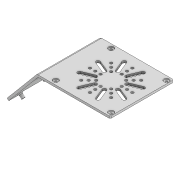
# Autodesk Inventor part: Electronics holder
Saved by Autodesk Inventor 2020 (Build 240168000, 168)
## iProperties
Created: 2021-10-18
Part Number: Electronics holder
Material: Generic
Document SubType Name: Modeling
Designer: ferrerx
Density: 1 g/cm^3
Appearance: Default
Author: ferrerx
Autodesk Inventor part; units mm, degrees
ref_plane "YZ Plane" through (0, 0, 0) normal (1, 0, 0) x (0, 1, 0)
ref_plane "XZ Plane" through (0, 0, 0) normal (0, 1, 0) x (-1, 0, 0)
sketch "Sketch1" plane through (0, 0, 0) normal (0, 1, 0) x (-1, 0, 0)
  line L0 (-52.25, 52.25) -> (52.25, 52.25) construction
  line L1 (52.25, 52.25) -> (52.25, -52.25) construction
  line L2 (52.25, -52.25) -> (-52.25, -52.25) construction
  line L3 (-52.25, -52.25) -> (-52.25, 52.25) construction
  line L4 (-52.25, 52.25) -> (52.25, -52.25) construction
  line L5 (52.25, 52.25) -> (-52.25, -52.25) construction
  line L6 (-80, 60) -> (80, 60)
  line L7 (80, 60) -> (80, -60)
  line L8 (80, -60) -> (-80, -60)
  line L9 (-80, -60) -> (-80, 60)
  line L10 (-80, 60) -> (80, -60) construction
  line L11 (80, 60) -> (-80, -60) construction
  circle A0 centre (52.25, 52.25) radius 2
  circle A1 centre (52.25, -52.25) radius 2
  circle A2 centre (-52.25, -52.25) radius 2
  circle A3 centre (-52.25, 52.25) radius 2
  point P0 (0, 0)
  dimension "d0" = 104.5
  dimension "d1" = 104.5
  dimension "d2" = 160
  dimension "d3" = 120
  dimension "d4" = 4
  dimension "d5" = 4
  dimension "d6" = 4
  dimension "d7" = 4
  constraints: 24 end point, 4 centre point, 4 coincident, 4 midpoint, 4 parallel, 2 horizontal, 2 perpendicular
  measures "d0" distance of L1.end L2.end
  measures "d1" distance of L0.end L1.end
  measures "d2" distance of L7.end L8.end
  measures "d3" distance of L6.end L7.end
  measures "d4" diameter of A0
  measures "d5" diameter of A1
  measures "d6" diameter of A3
  measures "d7" diameter of A2
extrude "Extrusion1" add sketch "Sketch1" along normal blind 4
sketch "Sketch2" plane through (0, 4, 0) normal (0, 1, 0) x (1, 0, 0)
  line L0 (-43.10961, -50) -> (-39.10961, -50)
  line L1 (-39.10961, -50) -> (-39.10961, 50)
  line L2 (-39.10961, 50) -> (-43.10961, 50)
  line L3 (-43.10961, 50) -> (-43.10961, -50)
  line L4 (-43.10961, -50) -> (-39.10961, 50) construction
  line L5 (-39.10961, -50) -> (-43.10961, 50) construction
  line L6 (0, 0) -> (-41.10961, 0) construction
  dimension "d10" = 4
  dimension "d11" = 100
  constraints: 14 end point, 2 horizontal, 2 midpoint, 2 parallel, 1 perpendicular
  measures "d10" distance of L1.end L2.end
  measures "d11" distance of L2.end L0.start
extrude "Extrusion2" [suppressed]
sketch "Sketch3" plane through (0, 4, 0) normal (0, 1, 0) x (1, 0, 0)
  circle A0 centre (0, 0) radius 2.5
  dimension "d14" = 5
  constraints: 1 centre point, 1 coincident
  measures "d14" diameter of A0
extrude "Extrusion3" cut sketch "Sketch3" against normal blind 4
pattern_linear "Rectangular Pattern1" count 5 spacing 10 along (1, 0, 0) of "Extrusion3"
pattern_circular "Circular Pattern1" count 8 over 360 about axis through (0, 4, 0) along (0, -1, 0) of "Extrusion3", "Rectangular Pattern1"
sketch "Sketch4" plane through (0, 4, 0) normal (0, 1, 0) x (1, 0, 0)
  line L0 (0, 0) -> (-19.859021, 47.943918) construction
  circle A0 centre (0, 0) radius 2.5
  line L1 (0, 0) -> (0, 50) construction
  line L2 (-8.905592, 21.5) -> (-17.604076, 42.5) construction
  line L3 (-5.672013, 22.839392) -> (-14.370498, 43.839392)
  line L4 (-20.837655, 41.160608) -> (-12.13917, 20.160608)
  arc A1 (-12.13917, 20.160608) -> (-5.672013, 22.839392) centre (-8.905592, 21.5) ccw
  arc A2 (-14.370498, 43.839392) -> (-20.837655, 41.160608) centre (-17.604076, 42.5) ccw
  point P0 (-13.254834, 32)
  dimension "d23" = 22.5
  dimension "d24" = 32
  dimension "d94" = 7
  constraints: 12 end point, 4 point on circle, 4 tangent, 2 centre point, 2 point on line, 1 midpoint, 1 parallel, 1 vertical
  measures "d23" angle of L0 L1
  measures "d24" vertical distance of L0.start point (-13.255, 32)
  measures "d94" distance between parallel lines of L4 L3
extrude "Extrusion4" cut sketch "Sketch4" against normal blind 4 contours A1 L4 A2 L3
pattern_circular "Circular Pattern2" count 8 over 360 about axis through (0, 4, 0) along (0, -1, 0) of "Extrusion4"
ref_plane "Work Plane1" through (-80, 4, -60) normal (0.7660444, -0.6427876, 0) x (0, 0, 1)
sketch "Sketch5" plane through (-80, 4, -60) normal (0.7660444, -0.6427876, 0) x (0, 0, 1)
  line L0 (1.217722, 0) -> (120, 0)
  line L1 (120, 0) -> (0, 0)
  line L2 (0, 0) -> (0, 90)
  line L3 (0, 90) -> (120, 90)
  line L4 (120, 90) -> (120, 0)
  line L5 (0, -102.846018) -> (0, 0)
  line L6 (0, 0) -> (120, 0)
  point P0 (60, -48.358831)
  point P1 (0, 2.294306)
  dimension "d31" = 90
  constraints: 10 end point, 2 collinear, 2 parallel, 1 horizontal, 1 perpendicular
  measures "d31" distance of L1.end L2.end
extrude "Extrusion5" add sketch "Sketch5" along normal blind 4
sketch "Sketch6" plane through (-80, 4, -60) normal (-0.7660444, 0.6427876, 0) x (0, 0, 1)
  line L0 (0, 0) -> (120, 0) projected
  line L1 (60, 0) -> (60, -90) construction
  line L2 (105, -12.5) -> (15, -12.5) construction
  line L3 (15, -12.5) -> (15, -77.5) construction
  line L4 (15, -77.5) -> (105, -77.5) construction
  line L5 (105, -77.5) -> (105, -12.5) construction
  line L6 (105, -12.5) -> (15, -77.5) construction
  line L7 (15, -12.5) -> (105, -77.5) construction
  circle A0 centre (105, -77.5) radius 1.5
  circle A1 centre (105, -12.5) radius 1.5
  circle A2 centre (15, -12.5) radius 1.5
  circle A3 centre (15, -77.5) radius 1.5
  point P0 (60, 48.358831)
  point P1 (60, -45)
  dimension "d34" = 65
  dimension "d35" = 90
  dimension "d36" = 3
  dimension "d37" = 3
  dimension "d38" = 3
  dimension "d39" = 3
  constraints: 14 end point, 4 centre point, 4 coincident, 4 midpoint, 2 parallel, 1 horizontal, 1 perpendicular, 1 vertical
  measures "d34" distance of L2.end L3.end
  measures "d35" distance of L2.start L2.end
  measures "d36" diameter of A3
  measures "d37" diameter of A2
  measures "d38" diameter of A1
  measures "d39" diameter of A0
extrude "Extrusion6" cut sketch "Sketch6" against normal blind 4
sketch "Sketch7" plane through (-80, 4, -60) normal (-0.7660444, 0.6427876, 0) x (0, 0, 1)
  line L0 (71.5, -36) -> (43.5, -36)
  line L1 (43.5, -36) -> (43.5, -22)
  line L2 (43.5, -22) -> (71.5, -22)
  line L3 (71.5, -22) -> (71.5, -36)
  line L4 (71.5, -36) -> (43.5, -22) construction
  line L5 (43.5, -36) -> (71.5, -22) construction
  circle A0 centre (28.8, -19.3) radius 5
  line L6 (35.5, -70.5) -> (18.5, -70.5)
  line L7 (18.5, -70.5) -> (18.5, -47.5)
  line L8 (18.5, -47.5) -> (35.5, -47.5)
  line L9 (35.5, -47.5) -> (35.5, -70.5)
  line L10 (35.5, -70.5) -> (18.5, -47.5) construction
  line L11 (18.5, -70.5) -> (35.5, -47.5) construction
  line L12 (120, -90) -> (0, -90) projected
  line L13 (102, -90) -> (18, -90)
  line L14 (18, -90) -> (18, -72)
  line L15 (18, -72) -> (102, -72)
  line L16 (102, -72) -> (102, -90)
  circle A1 centre (15, -12.5) radius 1.5 projected
  circle A2 centre (15, -77.5) radius 1.5 projected
  circle A3 centre (105, -77.5) radius 1.5 projected
  point P0 (60, 48.358831)
  point P1 (57.5, -29)
  point P2 (27, -59)
  point P3 (18, -90)
  dimension "d42" = 42.5
  dimension "d43" = 16.5
  dimension "d44" = 14
  dimension "d45" = 28
  dimension "d46" = 13.8
  dimension "d47" = 6.8
  dimension "d48" = 10
  dimension "d49" = 18.5
  dimension "d50" = 12
  dimension "d51" = 23
  dimension "d52" = 17
  dimension "d54" = 3
  dimension "d61" = 18
  dimension "d88" = 3
  constraints: 32 end point, 6 parallel, 4 midpoint, 3 horizontal, 3 perpendicular, 1 centre point, 1 point on line
  measures "d42" horizontal distance of point (57.5, -29) A1.centre
  measures "d43" vertical distance of point (57.5, -29) A1.centre
  measures "d44" distance of L2.end L0.start
  measures "d45" distance of L0.start L0.end
  measures "d46" horizontal distance of A0.centre A1.centre
  measures "d47" vertical distance of A1.centre A0.centre
  measures "d48" diameter of A0
  measures "d49" vertical distance of A2.centre point (27, -59)
  measures "d50" horizontal distance of A2.centre point (27, -59)
  measures "d51" distance of L6.end L7.end
  measures "d52" distance of L7.end L8.end
  measures "d54" distance from line of A3.centre L16
  measures "d61" distance of L13.end L14.end
  measures "d88" distance from line of A2.centre L14
extrude "Extrusion7" cut sketch "Sketch7" against normal blind 4 contours L0 L1 L2 L3 | A0 | L6 L7 L8 L9 | L12 L14 L15 L16
chamfer "Chamfer1" distance 2 angle 45 8 edges at (-136.3188, -66.2296, -60) (-136.3188, -66.2296, 60) (-80, 4, 0) (-78.1348, 0, 0) (80, 2, 60) (80, 2, -60) (-136.3188, -66.2296, 42) (-136.3188, -66.2296, -42)
fillet "Fillet1" radius 0.5 10 edges at (-101.6083, -24.8632, 11.5) (-101.6083, -24.8632, -16.5) (-92.6092, -14.1386, -16.5) (-92.6092, -14.1386, 11.5) (-123.7844, -51.2917, -24.5) (-123.7844, -51.2917, -41.5) (-109.0003, -33.6727, -24.5) (-109.0003, -33.6727, -41.5) (-124.7486, -52.4408, 42) (-124.7486, -52.4408, -42)
sketch "Sketch8" plane through (0, 4, 0) normal (0, 1, 0) x (1, 0, 0)
  line L0 (-76.134769, -60) -> (78, -60)
  line L1 (60, 60) -> (-47, 60)
  line L2 (-47, 60) -> (-47, -60)
  line L3 (-47, -60) -> (60, -60)
  line L4 (60, -60) -> (60, 60)
  point P0 (0, 0)
  point P1 (60, -60)
  constraints: 8 end point, 2 parallel, 1 horizontal, 1 perpendicular, 1 point on line
extrude "Extrusion8" [suppressed]
sketch "Sketch9" plane through (0, 0, 0) normal (0, -1, 0) x (1, 0, 0)
  circle A0 centre (-52.25, -52.25) radius 2 projected
  circle A1 centre (-52.25, -52.25) radius 2
  circle A2 centre (-52.25, -52.25) radius 4
  circle A3 centre (-52.25, 52.25) radius 2 projected
  circle A4 centre (-52.25, 52.25) radius 4
  circle A5 centre (52.25, 52.25) radius 2 projected
  circle A6 centre (52.25, 52.25) radius 4
  circle A7 centre (52.25, -52.25) radius 2 projected
  circle A8 centre (52.25, -52.25) radius 4
  point P0 (0, 0)
  dimension "d64" = 8
  dimension "d65" = 8
  dimension "d66" = 8
  dimension "d67" = 8
  constraints: 5 centre point, 5 coincident
  measures "d64" diameter of A2
  measures "d65" diameter of A4
  measures "d66" diameter of A6
  measures "d67" diameter of A8
sketch "Sketch10" plane through (-76.935822, 1.42885, -60) normal (0.7660444, -0.6427876, 0) x (0, 0, -1)
  circle A0 centre (-15, -12.5) radius 1.5 projected
  circle A1 centre (-15, -12.5) radius 3
  circle A2 centre (-105, -12.5) radius 1.5 projected
  circle A3 centre (-105, -12.5) radius 3
  circle A4 centre (-105, -77.5) radius 1.5 projected
  circle A5 centre (-105, -77.5) radius 3
  circle A6 centre (-15, -77.5) radius 1.5 projected
  circle A7 centre (-15, -77.5) radius 3
  point P0 (-60, 48.358831)
  dimension "d68" = 6
  dimension "d69" = 6
  dimension "d70" = 6
  dimension "d71" = 6
  constraints: 4 centre point, 4 coincident
  measures "d68" diameter of A5
  measures "d69" diameter of A7
  measures "d70" diameter of A1
  measures "d71" diameter of A3
extrude "Extrusion9" add sketch "Sketch10" along normal blind 8
fillet "Fillet2" radius 2 5 edges at (-128.6802, -60.2377, -45) (-124.8235, -55.6415, -45) (-126.7519, -57.9396, 48) (-84.9707, -8.1467, 48) (-84.9707, -8.1467, -42)
sketch "Sketch11" plane through (0, 4, 0) normal (0, 1, 0) x (1, 0, 0)
  line L0 (-76.134769, -60) -> (78, -60)
  line L1 (58, -60) -> (80, -60)
  line L2 (80, -60) -> (80, 60)
  line L3 (80, 60) -> (58, 60)
  line L4 (58, 60) -> (58, -60)
  line L5 (80, -58) -> (80, 58)
  point P0 (0, 0)
  dimension "d75" = 120
  dimension "d76" = 22
  constraints: 8 end point, 2 parallel, 1 collinear, 1 horizontal, 1 perpendicular, 1 point on line
  measures "d75" distance of L1.end L2.end
  measures "d76" distance between parallel lines of L2 L4
extrude "Extrusion10" cut sketch "Sketch11" against normal blind 12
chamfer "Chamfer2" distance 2 angle 45 2 edges at (58, 2, -60) (58, 2, 60)
sketch "Sketch12" plane through (0, 4, 0) normal (0, 1, 0) x (1, 0, 0)
  circle A0 centre (-52.25, -52.25) radius 2 projected
  circle A1 centre (-52.25, -52.25) radius 5
  circle A2 centre (-52.25, 52.25) radius 2 projected
  circle A3 centre (-52.25, 52.25) radius 5
  circle A4 centre (52.25, 52.25) radius 2 projected
  circle A5 centre (52.25, 52.25) radius 5
  circle A6 centre (52.25, -52.25) radius 2 projected
  circle A7 centre (52.25, -52.25) radius 5
  point P0 (0, 0)
  dimension "d82" = 10
  dimension "d83" = 10
  dimension "d84" = 10
  dimension "d85" = 10
  constraints: 4 centre point, 4 coincident
  measures "d82" diameter of A1
  measures "d83" diameter of A3
  measures "d84" diameter of A5
  measures "d85" diameter of A7
extrude "Extrusion11" cut sketch "Sketch12" against normal blind 2 contours A0 | A1 | A3 | A4 | A5 | A7
sketch "Sketch13" plane through (0, 4, 0) normal (0, 1, 0) x (1, 0, 0)
  circle A0 centre (0, 0) radius 15
  dimension "d89" = 30
  constraints: 1 centre point, 1 coincident
  measures "d89" diameter of A0
extrude "Extrusion12" add sketch "Sketch13" against normal blind 4
sketch "Sketch14" plane through (0, 4, 0) normal (0, 1, 0) x (1, 0, 0)
  line L0 (-76.134769, -60) -> (56, -60)
  line L1 (-43, -60) -> (58, -60)
  line L2 (58, -60) -> (58, 60)
  line L3 (58, 60) -> (-43, 60)
  line L4 (-43, 60) -> (-43, -60)
  point P0 (0, 0)
  constraints: 8 end point, 2 parallel, 1 horizontal, 1 perpendicular, 1 point on line
extrude "Extrusion13" [suppressed]
body "Solid1"
